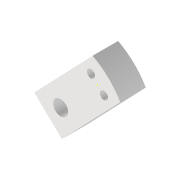
# Autodesk Inventor part: IM_Matchboxscope_Laserholder_2
Saved by Autodesk Inventor 2022 (Build 260153000, 153)
## iProperties
Created: 2023-05-17
Part Number: IM_Matchboxscope_Laserholder_2
Material: Generisch
Document SubType Name: Modeling
Designer: diederichbenedict
Density: 1 g/cm^3
Appearance: Vorgabe
Author: diederichbenedict
Autodesk Inventor part; units mm, degrees
ref_plane "YZ Plane" through (0, 0, 0) normal (1, 0, 0) x (0, 1, 0)
ref_plane "XZ Plane" through (0, 0, 0) normal (0, 1, 0) x (-1, 0, 0)
ref_plane "XY Plane" through (0, 0, 0) normal (0, 0, 1) x (1, 0, 0)
sketch "Skizze1" plane through (0, 0, 0) normal (0, 0, 1) x (1, 0, 0)
  circle A0 centre (2.5036, -2.4424) radius 1.4 construction
  circle A1 centre (-2.5484, 2.3924) radius 1.4 construction
  arc A2 (8.8953, -1.5488) -> (-1.9335, 8.8203) centre (-14.4319, -15.0709) ccw projected
  line L0 (-1.9335, 8.8203) -> (-8.8953, 1.5457) projected
  line L1 (-8.8953, 1.5457) -> (1.9365, -8.8203) projected
  line L2 (1.9365, -8.8203) -> (8.8953, -1.5488) projected
  arc A3 (-17.415, -14.7529) -> (-12.7255, -17.5384) centre (-14.4319, -15.0709) ccw projected
  line L3 (-8.8953, 1.5457) -> (-24.7975, -15.0712)
  line L4 (-24.7975, -15.0712) -> (-13.9657, -25.4371)
  line L5 (-13.9657, -25.4371) -> (1.9365, -8.8203)
  arc A4 (-13.2888, -12.8475) -> (-12.2085, -16.214) centre (-14.4319, -15.0709) ccw projected
  circle A5 centre (-14.4319, -15.0709) radius 2.95
  circle A6 centre (-2.5484, 2.3924) radius 1.6
  circle A7 centre (2.5036, -2.4424) radius 1.6
  point P0 (0, 0)
  dimension "d0" = 23
  dimension "d1" = 5.9
  dimension "d2" = 3.2
  dimension "d3" = 3.2
  constraints: 6 end point, 3 centre point, 3 coincident, 2 perpendicular
  measures "d0" distance between parallel lines of L4 L1
  measures "d1" diameter of A5
  measures "d2" diameter of A6
  measures "d3" diameter of A7
extrude "Extrusion1" add sketch "Skizze1" along normal blind 10
sketch "Skizze2" plane through (0, 0, 10) normal (0, 0, 1) x (1, 0, 0)
  point P0 (0, 0)
sketch "Skizze3" plane through (0, 0, 10) normal (0, 0, 1) x (1, 0, 0)
  point P0 (0, 0)
